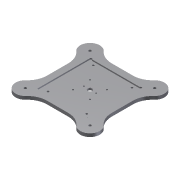
# Autodesk Inventor part: JointA0
Saved by Autodesk Inventor 2011 SP1 (Build 150282100, 282)
## iProperties
Created: 2012-10-15
Part Number: JointA0
Document SubType Name: Modeling
Designer: JohnHenry
Density: 1 g/cm^3
Author: JohnHenry
Autodesk Inventor part; units mm, degrees
ref_plane "YZ Plane" through (0, 0, 0) normal (1, 0, 0) x (0, 1, 0)
ref_plane "XZ Plane" through (0, 0, 0) normal (0, 1, 0) x (-1, 0, 0)
ref_plane "XY Plane" through (0, 0, 0) normal (0, 0, 1) x (1, 0, 0)
sketch "スケッチ1" plane through (0, 0, 0) normal (0, 0, 1) x (1, 0, 0)
  line L0 (-50, 50) -> (50, 50)
  line L1 (50, 50) -> (50, -50)
  line L2 (50, -50) -> (-50, -50)
  line L3 (-50, -50) -> (-50, 50)
  point P0 (0, 0)
  dimension "d0" = 100
  dimension "d1" = 100
  dimension "d2" = 50
  dimension "d3" = 50
  constraints: 8 end point, 2 parallel, 1 horizontal, 1 perpendicular
  measures "d0" distance of L2.end L0.start
  measures "d1" distance of L1.end L2.end
  measures "d2" distance from line of L3 point (0, 0)
  measures "d3" distance from line of L2 point (0, 0)
extrude "押し出し1" add sketch "スケッチ1" along normal blind 3
sketch "スケッチ2" plane through (0, 0, 3) normal (0, 0, 1) x (1, 0, 0)
  point P0 (0, 0)
  point P1 (0, 0)
  constraints: 1 coincident
hole "Hole1" at (0, 0, 3) direction (0, 0, -1) diameter 6 end through all counterbore diameter 7 counterbore depth 0.5
sketch "スケッチ3" plane through (0, 0, 3) normal (0, 0, 1) x (1, 0, 0)
  circle A0 centre (0, 0) radius 3.5 projected
  line L0 (50, 50) -> (50, -50) projected
  line L1 (-50, 50) -> (50, 50) projected
  line L2 (-50, -50) -> (-50, 50) projected
  line L3 (50, -50) -> (-50, -50) projected
  line L4 (-40.1, 40.1) -> (40.1, 40.1)
  line L5 (40.1, 40.1) -> (40.1, -40.1)
  line L6 (40.1, -40.1) -> (-40.1, -40.1)
  line L7 (-40.1, -40.1) -> (-40.1, 40.1)
  dimension "d13" = 80.2
  dimension "d14" = 80.2
  dimension "d15" = 40.1
  dimension "d16" = 40.1
  constraints: 8 end point, 2 parallel, 1 horizontal, 1 perpendicular
  measures "d13" distance of L4.start L4.end
  measures "d14" distance of L6.end L4.start
  measures "d15" distance from line of A0.centre L4
  measures "d16" distance from line of L7 A0.centre
extrude "押し出し2" add sketch "スケッチ3" along normal blind 2 contours L0 L3 L2 L1
sketch "スケッチ4" plane through (0, 0, 3) normal (0, 0, 1) x (1, 0, 0)
  circle A0 centre (0, 0) radius 3.5 projected
  point P0 (-29.9, 35)
  point P1 (-29.9, -35)
  point P2 (29.9, -35)
  point P3 (29.9, 35)
  dimension "d19" = 59.8
  dimension "d20" = 59.8
  dimension "d21" = 70
  dimension "d22" = 70
  dimension "d23" = 29.9
  dimension "d24" = 29.9
  dimension "d25" = 35
  measures "d19" distance of point (29.9, -35) point (-29.9, -35)
  measures "d20" distance of point (-29.9, 35) point (29.9, 35)
  measures "d21" distance of point (29.9, -35) point (29.9, 35)
  measures "d22" distance of point (-29.9, -35) point (-29.9, 35)
  measures "d23" horizontal distance of point (-29.9, 35) A0.centre
  measures "d24" horizontal distance of point (29.9, -35) A0.centre
  measures "d25" vertical distance of A0.centre point (29.9, 35)
hole "Hole2" at (29.9, -35, 3) at (-29.9, -35, 3) at (29.9, 35, 3) at (-29.9, 35, 3) direction (0, 0, -1) diameter 3 depth 8 tip angle 118
sketch "スケッチ5" plane through (0, 0, 0) normal (0, 0, -1) x (-1, 0, 0)
  circle A0 centre (-50, -50) radius 15
  circle A1 centre (-50, 50) radius 15
  circle A2 centre (50, -50) radius 15
  circle A3 centre (50, 50) radius 15
  dimension "d33" = 30
  dimension "d34" = 30
  dimension "d35" = 30
  dimension "d36" = 30
  constraints: 4 centre point, 4 coincident
  measures "d33" diameter of A0
  measures "d34" diameter of A1
  measures "d35" diameter of A2
  measures "d36" diameter of A3
extrude "押し出し3" add sketch "スケッチ5" against normal blind 5
fillet "フィレット1" radius 30 8 edges at (-35, 50, 2.5) (-50, 35, 2.5) (35, 50, 2.5) (50, 35, 2.5) (50, -35, 2.5) (35, -50, 2.5) (-35, -50, 2.5) (-50, -35, 2.5)
sketch "スケッチ6" plane through (0, 0, 0) normal (0, 0, -1) x (-1, 0, 0)
  arc A0 (60, 38.8197) -> (38.8197, 60) centre (50, 50) ccw projected
  arc A1 (-38.8197, 60) -> (-60, 38.8197) centre (-50, 50) ccw projected
  arc A2 (-60, -38.8197) -> (-38.8197, -60) centre (-50, -50) ccw projected
  arc A3 (38.8197, -60) -> (60, -38.8197) centre (50, -50) ccw projected
  constraints: 4 coincident
hole "Hole3" at (-50, -50, 0) at (50, -50, 0) at (50, 50, 0) at (-50, 50, 0) direction (0, 0, 1) diameter 4 depth 8 tip angle 118
sketch "スケッチ7" plane through (0, 0, 5) normal (0, 0, 1) x (1, 0, 0)
  arc A0 (-38.731, -40.1) -> (-40.1, -38.731) centre (-50, -50) ccw projected
  line L0 (-40.1, -38.731) -> (-40.1, 38.731) projected
  arc A1 (-40.1, 38.731) -> (-38.731, 40.1) centre (-50, 50) ccw projected
  line L1 (-38.731, 40.1) -> (38.731, 40.1) projected
  arc A2 (38.731, 40.1) -> (40.1, 38.731) centre (50, 50) ccw projected
  line L2 (40.1, 38.731) -> (40.1, -38.731) projected
  arc A3 (40.1, -38.731) -> (38.731, -40.1) centre (50, -50) ccw projected
  line L3 (38.731, -40.1) -> (-38.731, -40.1) projected
  circle A4 centre (-38.6, 40.1) radius 1.5
  line L4 (38.731, 40.1) -> (-38.731, 40.1) projected
  line L5 (0, 40.1) -> (0, -40.1)
  line L6 (40.1, 0) -> (-40.1, 0)
  circle A5 centre (38.6, 40.1) radius 1.5
  circle A6 centre (-38.6, -40.1) radius 1.5
  circle A7 centre (38.6, -40.1) radius 1.5
  line L7 (-40.1, 40.1) -> (40.1, 40.1)
  line L8 (40.1, 40.1) -> (40.1, -40.1)
  line L9 (40.1, -40.1) -> (-40.1, -40.1)
  line L10 (-40.1, -40.1) -> (-40.1, 40.1)
  point P0 (0, 0)
  dimension "d47" = 3
  dimension "d48" = 1.5
  constraints: 12 end point, 4 midpoint, 3 symmetric about line, 2 centre point, 2 horizontal alignment, 2 parallel, 2 point on line, 1 horizontal, 1 perpendicular, 7 other
  measures "d48" distance from line of L0 point (-38.6, 40.1)
extrude "押し出し4" cut sketch "スケッチ7" against normal up to surface (2 mm away) contours L9 A6 A0 | A0 A6 L3 | L3 A6 L9 | A6 L10 A0 | A7 A3 L3 | L3 L9 A7 | L10 A4 A1 | A3 A7 L9 | A3 L8 A7 | A4 L7 A1 | A1 L1 A4 | A4 L1 L7 | A5 L7 L1 | L1 A2 A5 | A2 A5 L8 | L7 A5 A2
sketch "スケッチ8" plane through (0, 0, 0) normal (0, 0, -1) x (-1, 0, 0)
  circle A0 centre (0, 0) radius 3 projected
  circle A1 centre (0, 0) radius 9.5
  point P0 (-9.5, 0)
  point P1 (9.5, 0)
  dimension "d51" = 19
  constraints: 2 point on circle, 1 centre point, 1 coincident
  measures "d51" diameter of A1
hole "Hole4" at (9.5, 0, 0) at (-9.5, 0, 0) direction (0, 0, 1) diameter 2.3 depth 8 tip angle 118
sketch "スケッチ9" plane through (0, 0, 0) normal (0, 0, -1) x (-1, 0, 0)
  circle A0 centre (0, 0) radius 3 projected
  line L0 (-16.459, -50) -> (16.459, -50) projected
  circle A1 centre (0, 0) radius 18.5
  line L1 (0, 0) -> (13.0815, 13.0815)
  line L2 (18.5, 0) -> (0, 0)
  point P0 (-13.0815, 13.0815)
  point P1 (-13.0815, -13.0815)
  point P2 (13.0815, -13.0815)
  dimension "d59" = 37
  dimension "d60" = 45
  dimension "d63" = 360
  constraints: 4 end point, 2 point on circle, 1 centre point, 1 coincident, 1 parallel, 5 other
  measures "d59" diameter of A1
  measures "d60" angle of L2 L1
hole "Hole5" at (-13.0815, 13.0815, 0) at (13.0815, 13.0815, 0) at (13.0815, -13.0815, 0) at (-13.0815, -13.0815, 0) direction (0, 0, 1) diameter 2.5 depth 8 tip angle 118
equation "\"d1\" = d0"
equation "\"d2\" = 0.5 * d0"
equation "\"d3\" = d2"
equation "\"d14\" = d13"
equation "\"d15\" = 0.5 * d13"
equation "\"d16\" = d15"
equation "\"d20\" = d19"
equation "\"d22\" = d21"
equation "\"d23\" = 0.5 * d19"
equation "\"d24\" = d23"
equation "\"d25\" = 0.5 * d21"
equation "\"d34\" = d33"
equation "\"d35\" = d33"
equation "\"d36\" = d33"
equation "\"d48\" = 0.5 * d47"
